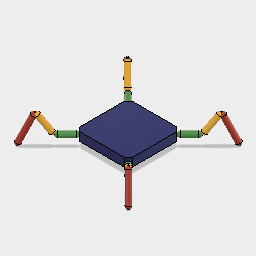
spider_simulator_model (Autodesk Fusion 360 design; units mm, degrees)
Autodesk Fusion 360 part; units mm, degrees
cylinder "CylinderPrimitive1" add diameter 10 height 25 placed x (1, 0, 0) y (0, 0, -1) z (0, 1, 0) at (0, 0, 0) makes body 1 in component "leg_1_Part_1"
sketch "Sketch3" plane through (0, 0, 0) normal (0, 0, 1) x (1, 0, 0)
  line L0 (0, 0) -> (0, 4.8)
  line L1 (0, 0) -> (5, 0)
  line L2 (0, 4.8) -> (1.4, 4.8)
  arc A0 (5, 0) -> (1.4, 4.8) centre (0, 0) ccw
  dimension "d11" = 10
  dimension "d12" = 4.8
  dimension "d13" = 5
  measures "d11" diameter of A0
  measures "d12" distance of L0.start L0.end
  measures "d13" distance of L0.start L1.end
revolve "Revolve1" add sketch "Sketch3" angle 360 about axis through (0, 0, 0) along (0, 1, 0) separate body makes body 2 in component "leg_1_Part_1_bottom"
revolve "Revolve1'" add sketch "Sketch3" angle 360 about axis through (0, 0, 0) along (0, 1, 0) separate body makes body 3 in component "leg_1_Part_1_top"
cylinder "CylinderPrimitive1'" add diameter 10 height 35 placed x (1, 0, 0) y (0, 0, -1) z (0, 1, 0) at (0, 0, 0) separate body makes body 4 in component "leg_1_Part_2"
revolve "Revolve1''" add sketch "Sketch3" angle 360 about axis through (0, 1.75, 0) along (0, 1, 0) separate body makes body 5 in component "leg_1_Part_2_bottom"
revolve "Revolve1'''" add sketch "Sketch3" angle 360 about axis through (0, 1.75, 0) along (0, 1, 0) separate body makes body 6 in component "leg_1_Part_2_top"
revolve "Revolve1''''" add sketch "Sketch3" angle 360 about axis through (0, 0, 0) along (0, 1, 0) separate body makes body 7 in component "leg_1_part_3_bottom"
cylinder "CylinderPrimitive1''" add diameter 10 height 50 placed x (1, 0, 0) y (0, 0, -1) z (0, 1, 0) at (0, 0, 0) separate body makes body 8
copy_body "Body->Comp1" bodies 8 removing the originals makes body 9 in component "leg_1_part_3"
revolve "Revolve1'''''" add sketch "Sketch3" angle 360 about axis through (0, 1.75, 0) along (0, 1, 0) separate body makes body 10 in component "leg_1_part_3_top"
ref_plane "WorkPlane1" through (0, 0, 0) normal (0, 1, 0) x (0, 0, 1)
sketch "Sketch7" plane through (0, 0, 0) normal (0, 1, 0) x (1, 0, 0)
  line L0 (50, -50) -> (-50, -50)
  line L1 (-50, -50) -> (-50, 50)
  line L2 (-50, 50) -> (50, 50)
  line L3 (50, 50) -> (50, -50)
  line L4 (50, -50) -> (-50, 50) construction
  line L5 (-50, -50) -> (50, 50) construction
  dimension "d185" = 100
  dimension "d186" = 100
  measures "d185" distance of L1.end L2.end
  measures "d186" distance of L0.end L1.end
extrude "Extrude1" add sketch "Sketch7" along normal mid plane 16 separate body makes body 11
chamfer "Chamfer1" distance 8 angle 45 1 edges at (50, 0, 50) on bodies 11
chamfer "Chamfer2" distance 8 angle 45 1 edges at (50, 0, -50) on bodies 11
chamfer "Chamfer3" distance 8 angle 45 1 edges at (-50, 0, 50) on bodies 11
chamfer "Chamfer4" distance 8 angle 45 1 edges at (-50, 0, -50) on bodies 11
copy_body "Body->Comp2" bodies 11 removing the originals makes body 12 in component "Body"
component "leg_1_Part_1" placed x (0.694395, 0, -0.719594) y (-0.719594, 0, -0.694395) z (0, 1, 0) at (-49.4541, 0, -49.3331)
component "leg_1_Part_2" placed x (0.694395, 0, -0.719594) y (0.412742, -0.819152, 0.398289) z (-0.589457, -0.573576, -0.568815) at (-87.3251, 32.6023, -85.878)
component "leg_1_part_3" placed x (0.304114, -0.906308, 0.293464) y (0.652174, 0.422618, 0.629336) z (-0.694395, 0, 0.719594) at (-125.0454, 13.3747, -122.2773)
component "Body" placed x (1, 0, 0) y (0, 1, 0) z (0, 0, 1) at (0, 0, 0)
component "leg_1_Part_1" placed x (0, 1, 0) y (0.707107, 0, -0.707107) z (-0.707107, 0, -0.707107) at (-67.0718, 0, 67.0718)
component "leg_1_Part_1" placed x (0, 1, 0) y (-0.707107, 0, -0.707107) z (-0.707107, 0, 0.707107) at (67.0718, 0, 67.0718)
component "leg_1_Part_1" placed x (0, 1, 0) y (-0.707107, 0, 0.707107) z (0.707107, 0, 0.707107) at (67.0718, 0, -67.0718)
component "leg_1_Part_2" placed x (0.579228, 0.573576, -0.579228) y (0.40558, -0.819152, -0.40558) z (-0.707107, 0, -0.707107) at (-86.608, 32.6023, 86.608)
component "leg_1_Part_2" placed x (-0.579228, 0.573576, -0.579228) y (-0.40558, -0.819152, -0.40558) z (-0.707107, 0, 0.707107) at (86.608, 32.6023, 86.608)
component "leg_1_Part_2" placed x (-0.579228, 0.573576, 0.579228) y (-0.40558, -0.819152, 0.40558) z (0.707107, 0, 0.707107) at (86.608, 32.6023, -86.608)
component "leg_1_part_3" placed x (-0.640856, -0.422618, -0.640856) y (-0.298836, 0.906308, -0.298836) z (0.707107, 0, -0.707107) at (104.931, -13.1315, 104.931)
component "leg_1_part_3" placed x (-0.640856, -0.422618, 0.640856) y (-0.298836, 0.906308, 0.298836) z (-0.707107, 0, -0.707107) at (104.931, -13.1315, -104.931)
component "leg_1_part_3" placed x (0.640856, -0.422618, -0.640856) y (0.298836, 0.906308, -0.298836) z (0.707107, 0, 0.707107) at (-104.931, -13.1315, 104.931)
component "leg_1_Part_1_bottom" placed x (1, 0, 0) y (0, 1, 0) z (0, 0, 1) at (0, 25, 0) in component "leg_1_Part_1"
component "leg_1_Part_1_top" placed x (1, 0, 0) y (0, -1, 0) z (0, 0, -1) at (0, 0, 0) in component "leg_1_Part_1"
component "leg_1_Part_2_bottom" placed x (1, 0, 0) y (0, -1, 0) z (0, 0, -1) at (0, 0, 0) in component "leg_1_Part_2"
component "leg_1_Part_2_top" placed x (1, 0, 0) y (0, 1, 0) z (0, 0, 1) at (0, 35, 0) in component "leg_1_Part_2"
component "leg_1_part_3_top" placed x (1, 0, 0) y (0, 1, 0) z (0, 0, 1) at (0, 50, 0) in component "leg_1_part_3"
component "leg_1_part_3_bottom" placed x (1, 0, 0) y (0, -1, 0) z (0, 0, -1) at (0, 0, 0) in component "leg_1_part_3"
